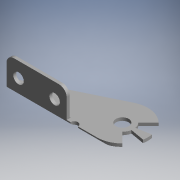
# Autodesk Inventor part: MHPUS306-Ab_fixed_left
Saved by Autodesk Inventor 2017.3 (Build 213256000, 256)
## iProperties
Part Number: MHPUS306-Ab_fixed_left
Material: Generic
Catalog Web Link: www.cadenas.de
Description: MHPUS_b_fixed_left-Cable Carriers Flap Open - Close Type
Vendor: MISUMI
Document SubType Name: Modeling
Designer: partserver
Manufacturer: MISUMI
Mass: 4.26247 g
Surface Area: 48.7006 cm^2
Volume: 4.26247 cm^3
Density: 1 g/cm^3
Appearance: PSOLRGB-192-192-192
Category: PARTsolutions
Company: MISUMI
Title: MHPUS306-Ab_fixed_left
Author: Cadenas PARTsolutions
Comments: Cable Carriers Flap Open - Close Type
PSOL_IDENT_0: {$CADENAS_DATA\23d-libs\misumi\metric\07_slide_rails\mhpus_bracket_fixed_left.prj},198 {VTYP=3D},{NB=
PSOL_IDENT_1: MHPUS306-Ab_fixed_left},{LINA=MHPUS306-Ab_fixed_left},{NN=MHPUS_b_fixed_left},{DATE=30.06.2021 12:53
PSOL_IDENT_2: :59},{GEOMDATE=01.09.2009 09:03:00},{VERSION=},{LINEID=80},{WBVAR=AD},{WBNUMERIC=}  {NB=MHPUS306-Ab_
PSOL_IDENT_3: fixed_left},{LINA=MHPUS306-Ab_fixed_left},{KT=DUMMY},{PN=MHPUS306-A},{NO=306},{MAT=Low Carbon Steel}
PSOL_IDENT_4: ,{ST=Trivalent Bright Chromate Plating},{AD=A},{ADALG= 'A', 'Outer circumference', 'B', 'Inner circu
PSOL_IDENT_5: mference' },{HH=34},{F=40},{T=24},{J=20},{N=7.0},{LL=60},{P1F=35.6},{P2F=55.6},{P1FX=32},{P2FX=52},{
PSOL_IDENT_6: R4=8.000},{R1=2.000},{R2=5.000},{R24=35.000},{R25=10.000},{R26=7.500},{END=1}
NB: MHPUS306-Ab_fixed_left
NN: MHPUS_b_fixed_left
NT: Cable Carriers Flap Open - Close Type
NBSYN: $PN.b_fixed_left
LINA: MHPUS306-Ab_fixed_left
CATALOG: Misumi
PN: MHPUS306-A
NO: 306
MAT: Low Carbon Steel
ST: Trivalent Bright Chromate Plating
AD: Outer circumference
HH: 34
F: 40
T: 24
J: 20
N: 7
LL: 60
P1F: 35.6
P2F: 55.6
P1FX: 32
P2FX: 52
R4: 8
R1: 2
R2: 5
R24: 35
R25: 10
R26: 7.5
SUPPLIER: MISUMI
ARTICLENO: MHPUS306-Ab_fixed_left
BOMINFO: MHPUS306-Ab_fixed_left
CREATOR: CADENAS GmbH
Autodesk Inventor part; units mm, degrees
sketch "Sketch_1" plane through (0, 0, 0) normal (0, 0, 1) x (1, 0, 0)
  arc A0 (-16.7417, 19.952) -> (-16.7417, 14.048) centre (0, 17) ccw
  line L0 (-16.7417, 14.048) -> (-7.3861, 15.6976)
  arc A1 (-7.3861, 15.6976) -> (-5.3033, 11.6967) centre (0, 17) ccw
  line L1 (-5.3033, 11.6967) -> (-12.0208, 4.9792)
  arc A2 (-12.0208, 4.9792) -> (0, 0) centre (0, 17) ccw
  line L2 (0, 0) -> (60, 0)
  line L3 (60, 0) -> (60, 4.67)
  arc A3 (60, 4.67) -> (58.0834, 7.7293) centre (56.6, 4.67) ccw
  line L4 (58.0834, 7.7293) -> (7.4171, 32.2966)
  arc A4 (7.4171, 32.2966) -> (-12.0208, 29.0208) centre (0, 17) ccw
  line L5 (-12.0208, 29.0208) -> (-5.3033, 22.3033)
  arc A5 (-5.3033, 22.3033) -> (-7.3861, 18.3024) centre (0, 17) ccw
  line L6 (-7.3861, 18.3024) -> (-16.7417, 19.952)
  circle A6 centre (0, 17) radius 4.25
  constraints: 14 end point, 12 point on circle, 7 centre point
extrude "Extrusion1" add sketch "Sketch_1" against normal blind 20
sketch "Sketch_2" plane through (0, 0, 0) normal (1, 0, 0) x (0, 1, 0)
  line L0 (39, 5) -> (-5, 5)
  line L1 (-5, 5) -> (-5, -25)
  line L2 (-5, -25) -> (39, -25)
  line L3 (39, -25) -> (39, 5)
  arc A0 (2, 0) -> (0, -2) centre (2, -2) ccw
  line L4 (0, -2) -> (0, -20)
  line L5 (0, -20) -> (2, -20)
  line L6 (2, -20) -> (2, -3)
  arc A1 (3, -2) -> (2, -3) centre (3, -3) ccw
  line L7 (3, -2) -> (34, -2)
  line L8 (34, -2) -> (34, 0)
  line L9 (34, 0) -> (2, 0)
  constraints: 20 end point, 4 point on circle, 2 centre point
extrude "Extrusion2" cut sketch "Sketch_2" along normal mid plane 120
sketch "Sketch_3" plane through (0, 0, 0) normal (0, 1, 0) x (-1, 0, 0)
  line L0 (22, -25) -> (22, 5)
  line L1 (22, 5) -> (-65, 5)
  line L2 (-65, 5) -> (-65, -25)
  line L3 (-65, -25) -> (22, -25)
  line L4 (17, -2) -> (17, 0)
  line L5 (17, 0) -> (-60, 0)
  line L6 (-60, 0) -> (-60, -15)
  arc A0 (-60, -15) -> (-55, -20) centre (-55, -15) ccw
  line L7 (-55, -20) -> (-25, -20)
  arc A1 (-25, -20) -> (-20, -15) centre (-25, -15) ccw
  line L8 (-20, -15) -> (-20, -2)
  line L9 (-20, -2) -> (17, -2)
  constraints: 20 end point, 4 point on circle, 2 centre point
extrude "Extrusion3" cut sketch "Sketch_3" along normal blind 34
sketch "Sketch4" plane through (20, 0, -2) normal (0, -1, 0) x (1, 0, 0)
  point P0 (8, -8)
hole "Hole1" at (28, 0, -10) direction (0, 1, 0) diameter 7 depth 2
sketch "Sketch5" plane through (20, 0, -2) normal (0, -1, 0) x (1, 0, 0)
  point P0 (32, -8)
hole "Hole2" at (52, 0, -10) direction (0, 1, 0) diameter 7 depth 2
sketch "Sketch_7" plane through (0, 0, 0) normal (0, 0, 1) x (1, 0, 0)
  circle A0 centre (15, 0) radius 2.5
  constraints: 1 centre point
extrude "Extrusion4" cut sketch "Sketch_7" against normal blind 20
ref_plane "fix_end_l_XY" through (0, 17, 0) normal (0, 0, 1) x (1, 0, 0)
ref_plane "fix_end_l_YZ" through (0, 17, 0) normal (1, 0, 0) x (0, 1, 0)
ref_plane "fix_end_l_ZX" through (0, 17, 0) normal (0, 1, 0) x (0, 0, 1)
ref_plane "free_end_l_XY" through (0, 17, -2) normal (0, 0, 1) x (1, 0, 0)
ref_plane "free_end_l_YZ" through (0, 17, -2) normal (1, 0, 0) x (0, 1, 0)
ref_plane "free_end_l_ZX" through (0, 17, -2) normal (0, 1, 0) x (0, 0, 1)
ref_plane "l_to_r_XY" through (0, 17, -26) normal (0, 0, 1) x (1, 0, 0)
ref_plane "l_to_r_YZ" through (0, 17, -26) normal (1, 0, 0) x (0, 1, 0)
ref_plane "l_to_r_ZX" through (0, 17, -26) normal (0, 1, 0) x (0, 0, 1)
ref_plane "to_clip1_XY" through (0, 17, -10) normal (1, 0, 0) x (0, 0, -1)
ref_plane "to_clip1_YZ" through (0, 17, -10) normal (0, 0, -1) x (0, 1, 0)
ref_plane "to_clip1_ZX" through (0, 17, -10) normal (0, 1, 0) x (1, 0, 0)
body "Solid1"
